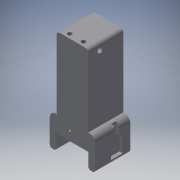
# Autodesk Inventor part: Part1
Saved by Autodesk Inventor 2016 (Build 200138000, 138)
## iProperties
Created: 2016-11-19
Part Number: Part1
Material: Generic
Document SubType Name: Modeling
Designer: Juraj
Density: 1 g/cm^3
Appearance: Default
Author: Juraj
Autodesk Inventor part; units mm, degrees
ref_plane "YZ Plane" through (0, 0, 0) normal (1, 0, 0) x (0, 1, 0)
ref_plane "XZ Plane" through (0, 0, 0) normal (0, 1, 0) x (-1, 0, 0)
ref_plane "XY Plane" through (0, 0, 0) normal (0, 0, 1) x (1, 0, 0)
sketch "Sketch1" plane through (0, 0, 0) normal (0, 1, 0) x (-1, 0, 0)
  line L0 (7.9968, 14.4905) -> (-11.0032, 14.4905)
  line L1 (-11.0032, 14.4905) -> (-11.0032, -38.5095)
  line L2 (-11.0032, -38.5095) -> (7.9968, -38.5095)
  line L3 (7.9968, -38.5095) -> (7.9968, 14.4905)
  point P0 (0, 0)
  dimension "d0" = 19
  dimension "d1" = 53
  constraints: 8 end point, 2 parallel, 1 horizontal, 1 perpendicular
  measures "d0" distance of L0.start L0.end
  measures "d1" distance of L2.end L0.start
extrude "Extrusion1" add sketch "Sketch1" along normal blind 1
sketch "Sketch2" plane through (0, 1, 0) normal (0, 1, 0) x (1, 0, 0)
  line L0 (9.0032, -13.4905) -> (-5.9968, -13.4905)
  line L1 (-5.9968, -13.4905) -> (-5.9968, 37.5095)
  line L2 (-5.9968, 37.5095) -> (9.0032, 37.5095)
  line L3 (9.0032, 37.5095) -> (9.0032, -13.4905)
  line L4 (11.0032, -14.4905) -> (11.0032, 38.5095) projected
  line L5 (-7.9968, -14.4905) -> (11.0032, -14.4905) projected
  line L6 (-7.9968, 38.5095) -> (-7.9968, -14.4905) projected
  line L7 (11.0032, 38.5095) -> (-7.9968, 38.5095) projected
  point P0 (0, 0)
  dimension "d4" = 2
  dimension "d5" = 1
  dimension "d6" = 2
  dimension "d7" = 1
  constraints: 8 end point, 2 parallel, 1 horizontal, 1 perpendicular
  measures "d4" distance between parallel lines of L4 L3
  measures "d5" distance between parallel lines of L5 L0
  measures "d6" distance between parallel lines of L6 L1
  measures "d7" distance between parallel lines of L7 L2
extrude "Extrusion2" add sketch "Sketch2" along normal blind 18
sketch "Sketch5" plane through (11.0032, 0, -38.5095) normal (0, 0, -1) x (-1, 0, 0)
  line L0 (17, 1) -> (2, 1) projected
  line L1 (9.5, 1) -> (9.5, 6)
  line L2 (9.5, 6) -> (9.5, 13.4)
  circle A0 centre (9.5, 13.4) radius 2
  line L3 (2, 1) -> (2, 19) projected
  line L4 (17, 1) -> (17, 19) projected
  point P0 (11.0032, 0)
  dimension "d28" = 5
  dimension "d29" = 7.4
  dimension "d30" = 4
  dimension "d31" = 7.5
  dimension "d32" = 7.5
  constraints: 4 end point, 1 centre point, 1 coincident, 1 midpoint, 1 perpendicular, 1 vertical
  measures "d28" distance of L1.start L1.end
  measures "d29" distance of L1.end L2.end
  measures "d30" diameter of A0
  measures "d31" distance between parallel lines of L3 L1
  measures "d32" distance between parallel lines of L4 L1
extrude "Extrusion3" cut sketch "Sketch5" against normal blind 13
sketch "Sketch6" plane through (-5.9968, 1, -37.5095) normal (0, 0, 1) x (1, 0, 0)
  circle A0 centre (7.5, 12.4) radius 2 projected
  circle A1 centre (7.5, 12.4) radius 3.55
  line L0 (3.9514, 12.5) -> (0, 12.5)
  line L1 (0, 0) -> (0, 18) projected
  line L2 (11.0486, 12.5) -> (15, 12.5)
  line L3 (15, 0) -> (15, 18) projected
  line L4 (15, 12.5) -> (15, 0)
  line L5 (15, 0) -> (0, 0) projected
  line L6 (15, 0) -> (0, 0)
  line L7 (0, 0) -> (0, 12.5)
  line L8 (3.9514, 12.5) -> (0, 12.5)
  line L9 (0, 12.5) -> (0, 18)
  line L10 (0, 18) -> (3.9514, 18)
  line L11 (3.9514, 18) -> (3.9514, 12.5)
  line L12 (11.0486, 12.5) -> (15, 12.5)
  line L13 (15, 12.5) -> (15, 18)
  line L14 (15, 18) -> (11.0486, 18)
  line L15 (11.0486, 18) -> (11.0486, 12.5)
  point P0 (5.9968, -1)
  dimension "d35" = 7.1
  constraints: 26 end point, 4 parallel, 4 point on line, 3 collinear, 3 horizontal, 2 perpendicular, 2 point on circle, 1 centre point, 1 coincident
  measures "d35" diameter of A1
extrude "Extrusion4" add sketch "Sketch6" along normal blind 3.5 contours A1 L2 L3 L5 L1 L0 | L15 L14 L3 L2 | L0 L1 L10 L11
sketch "Sketch7" plane through (9.0032, 1, 13.4905) normal (0, 0, -1) x (-1, 0, 0)
  circle A0 centre (7.5, 12.4) radius 2 projected
  circle A1 centre (7.5, 12.4) radius 2
  line L0 (15, 0) -> (0, 0) projected
  line L1 (0, 0) -> (15, 0)
  line L2 (15, 0) -> (15, 18) projected
  circle A2 centre (7.5, 12.4) radius 3.55
  line L3 (11.0486, 12.5) -> (15, 12.5)
  line L4 (15, 12.5) -> (15, 0)
  line L5 (17, -1) -> (-2, -1) projected
  line L6 (15, 0) -> (0, 0)
  line L7 (0, 0) -> (0, 12.5)
  line L8 (0, 12.5) -> (3.9514, 12.5)
  line L9 (0, 18) -> (15, 18) projected
  line L10 (3.9514, 12.5) -> (0, 12.5)
  line L11 (0, 12.5) -> (0, 18)
  line L12 (0, 18) -> (3.9514, 18)
  line L13 (3.9514, 18) -> (3.9514, 12.5)
  line L14 (11.0486, 12.5) -> (15, 12.5)
  line L15 (15, 12.5) -> (15, 18)
  line L16 (15, 18) -> (11.0486, 18)
  line L17 (11.0486, 18) -> (11.0486, 12.5)
  point P0 (9.0032, -1)
  dimension "d40" = 7.1
  constraints: 28 end point, 5 equal length, 5 perpendicular, 3 horizontal, 2 centre point, 2 coincident, 2 point on circle, 2 point on line
  measures "d40" diameter of A2
extrude "Extrusion5" add sketch "Sketch7" along normal blind 3.5 contours L0 L7 L8 A2 L3 L2 | L3 L17 L9 L2 | L11 L9 L13 L8
sketch "Sketch9" plane through (0, 1, 0) normal (0, 1, 0) x (1, 0, 0)
  line L0 (-5.9968, -9.9905) -> (9.0032, -9.9905) projected
  line L1 (9.0032, -9.9905) -> (9.0032, -7.9905)
  line L2 (9.0032, -9.9905) -> (9.0032, 34.0095) projected
  line L3 (9.0032, -7.9905) -> (-5.9968, -7.9905)
  line L4 (-5.9968, 34.0095) -> (-5.9968, -9.9905) projected
  line L5 (9.0032, 34.0095) -> (9.0032, 33.0095)
  line L6 (9.0032, 33.0095) -> (-5.9968, 33.0095)
  line L7 (-5.9968, 33.0095) -> (-5.9968, 34.0095)
  line L8 (9.0032, 34.0095) -> (-5.9968, 34.0095)
  line L9 (-5.9968, 33.0095) -> (-5.9968, 34.0095)
  line L10 (9.0032, 34.0095) -> (5.0518, 34.0095) projected
  line L11 (9.0032, 34.0095) -> (-5.9968, 34.0095)
  line L12 (-5.9968, -13.4905) -> (-5.9968, 37.5095) projected
  point P0 (0, 0)
  dimension "d46" = 2
  dimension "d47" = 1
  constraints: 16 end point, 4 point on line, 3 perpendicular, 2 collinear, 1 horizontal
  measures "d46" distance of L0.end L1.end
  measures "d47" distance of L2.end L5.end
extrude "Extrusion7" add sketch "Sketch9" along normal blind 18 contours L4 L3 L1 L0 | L4 L8 L2 L6
sketch "Sketch12" plane through (0, 1, 0) normal (0, 1, 0) x (1, 0, 0)
  line L0 (9.0032, 33.0095) -> (-5.9968, 33.0095) projected
  line L1 (-5.9968, -7.9905) -> (-4.6968, -7.9905)
  line L2 (-4.6968, -7.9905) -> (-4.6968, 33.0095)
  line L3 (-5.9968, 33.0095) -> (-5.9968, -7.9905) projected
  line L4 (-5.9968, -7.9905) -> (-5.9968, 33.0095)
  line L5 (-5.9968, 33.0095) -> (-4.6968, 33.0095)
  line L6 (-5.9968, 33.0095) -> (-4.6968, 33.0095)
  line L7 (5.0518, 34.0095) -> (-2.0454, 34.0095) projected
  line L8 (9.0032, -7.9905) -> (7.7032, -7.9905)
  line L9 (7.7032, -7.9905) -> (7.7032, 33.0095)
  line L10 (-5.9968, 33.0095) -> (9.0032, 33.0095) projected
  line L11 (9.0032, 33.0095) -> (7.7032, 33.0095)
  line L12 (9.0032, 33.0095) -> (9.0032, -7.9905) projected
  line L13 (9.0032, -7.9905) -> (9.0032, 33.0095)
  line L14 (9.0032, 33.0095) -> (7.7032, 33.0095)
  point P0 (0, 0)
  point P1 (31.8085, 33.0095)
  point P2 (9.0032, 34.0095)
  point P3 (-5.9968, 34.0095)
  dimension "d61" = 1.3
  dimension "d153" = 1.3
  constraints: 20 end point, 4 perpendicular, 3 point on line, 2 collinear, 1 vertical
  measures "d61" distance of L1.start L1.end
  measures "d153" distance between parallel lines of L12 L9
extrude "Extrusion9" add sketch "Sketch12" along normal blind 18
sketch "Sketch10" plane through (9.0032, 19, -34.0095) normal (0, 0, -1) x (-1, 0, 0)
  circle A0 centre (7.5, -5.6) radius 2 projected
  circle A1 centre (7.5, -5.6) radius 2
  point P0 (9.0032, -19)
  constraints: 1 centre point, 1 coincident
extrude "Extrusion8" cut sketch "Sketch10" against normal blind 46
sketch "Sketch13" plane through (0, 1, 0) normal (0, 1, 0) x (1, 0, 0)
  line L0 (3.5032, -6.9905) -> (-0.4968, -6.9905)
  line L1 (-4.6968, -7.9905) -> (-4.6968, 33.0095) projected
  line L2 (-4.6968, 19.3095) -> (-3.1968, 19.3095)
  line L3 (-3.1968, 19.3095) -> (-3.1968, 21.3095)
  line L4 (-3.1968, 21.3095) -> (-4.6968, 21.3095)
  line L5 (7.7032, 19.3095) -> (6.2032, 19.3095)
  line L6 (6.2032, 19.3095) -> (6.2032, 21.3095)
  line L7 (6.2032, 21.3095) -> (7.7032, 21.3095)
  line L8 (-0.4968, -7.9905) -> (3.5032, -7.9905) projected
  line L9 (3.5032, -7.9905) -> (3.5032, -6.9905)
  line L10 (-0.4968, -7.9905) -> (-0.4968, -6.9905)
  line L11 (3.5032, -7.9905) -> (-0.4968, -7.9905)
  line L12 (7.7032, -7.9905) -> (-4.6968, -7.9905) projected
  line L13 (7.7032, 19.3095) -> (7.7032, 21.3095)
  line L14 (7.7032, 33.0095) -> (7.7032, -7.9905) projected
  point P0 (0, 0)
  dimension "d76" = 26.3
  dimension "d77" = 2
  dimension "d78" = 1.5
  dimension "d79" = 1.5
  dimension "d89" = 1
  dimension "d169" = 0
  dimension "d170" = 2
  constraints: 22 end point, 5 perpendicular, 5 point on line, 2 collinear, 1 parallel
  measures "d76" distance between parallel lines of L0 L5
  measures "d77" distance of L5.end L6.end
  measures "d78" distance of L3.end L4.end
  measures "d79" distance of L6.end L7.end
  measures "d89" distance of L8.end L0.start
  measures "d169" distance between parallel lines of L14 L13
  measures "d170" distance of L5.start L7.end
extrude "Extrusion10" add sketch "Sketch13" along normal blind 8
sketch "Sketch11" plane through (0, 1, 0) normal (0, 1, 0) x (1, 0, 0)
  line L0 (7.5032, -6.9905) -> (-4.4968, -6.9905)
  line L1 (-4.4968, -6.9905) -> (-4.4968, 19.0095)
  line L2 (-4.4968, 19.0095) -> (7.5032, 19.0095)
  line L3 (7.5032, 19.0095) -> (7.5032, -6.9905)
  line L4 (-5.9968, -7.9905) -> (-5.9968, 33.0095) projected
  line L5 (1.5032, 19.0095) -> (5.5033, 19.0095)
  line L6 (5.5033, 19.0095) -> (5.5033, 28.0095)
  line L7 (5.5033, 28.0095) -> (-2.4967, 28.0095)
  line L8 (-2.4967, 28.0095) -> (-2.4967, 19.0095)
  line L9 (5.5033, 23.0095) -> (-2.4967, 23.0095)
  line L10 (-2.4967, 23.0095) -> (-2.4967, 32.0095)
  line L11 (-2.0454, 37.5095) -> (-2.0454, 34.0095) projected
  line L12 (9.0032, -7.9905) -> (-5.9968, -7.9905) projected
  line L13 (3.5032, -6.9905) -> (-0.4968, -6.9905) projected
  point P0 (0, 0)
  point P1 (-2.0468, 37.5095)
  point P2 (-2.0468, 34.0095)
  dimension "d52" = 12
  dimension "d53" = 1.5
  dimension "d54" = 9
  dimension "d55" = 8
  dimension "d56" = 4
  dimension "d57" = 9
  dimension "d59" = 26
  dimension "d83" = 0
  constraints: 20 end point, 5 perpendicular, 4 point on line, 2 horizontal, 2 vertical, 1 midpoint, 1 other
  measures "d52" distance of L0.start L0.end
  measures "d53" distance between parallel lines of L4 L1
  measures "d54" distance of L5.end L6.end
  measures "d55" distance of L6.end L7.end
  measures "d56" distance between parallel lines of L2 L9
  measures "d57" distance of L9.end L10.end
  measures "d59" distance of L0.end L1.end
  measures "d83" distance between parallel lines of L13 L0
fillet "Fillet1" radius 2 2 edges at (-0.4968, 9, 7.4905) (3.5032, 9, 7.4905)
fillet "Fillet2" radius 0.5 2 edges at (6.2032, 9, -20.3095) (-3.1968, 9, -20.3095)
sketch "Sketch16" plane through (11.0032, 0, 14.4905) normal (1, 0, 0) x (0, 0, -1)
  circle A0 centre (4, 7) radius 1.5
  line L0 (53, 0) -> (0, 0) projected
  line L1 (0, 0) -> (0, 19) projected
  point P0 (14.4905, 0)
  point P1 (52, 0)
  dimension "d84" = 3
  dimension "d85" = 7
  dimension "d86" = 4
  constraints: 1 centre point
  measures "d84" diameter of A0
  measures "d85" distance from line of L0 A0.centre
  measures "d86" distance from line of L1 A0.centre
extrude "Extrusion12" cut sketch "Sketch16" against normal blind 19
sketch "Sketch20" plane through (11.0032, 0, 14.4905) normal (1, 0, 0) x (0, 0, -1)
  line L0 (0, 19) -> (53, 19) projected
  line L1 (43, 19) -> (62, 19)
  line L2 (62, 19) -> (62, 0)
  line L3 (62, 0) -> (43, 0)
  line L4 (43, 0) -> (43, 19)
  line L5 (53, 15.4) -> (53, 11.4) projected
  line L6 (53, 0) -> (53, 19) projected
  point P0 (14.4905, 0)
  dimension "d106" = 9
  dimension "d107" = 10
  constraints: 8 end point, 2 parallel, 1 horizontal, 1 perpendicular, 1 point on line
  measures "d106" distance between parallel lines of L5 L2
  measures "d107" distance between parallel lines of L6 L4
extrude "Extrusion15" add sketch "Sketch20" along normal blind 4
sketch "Sketch21" plane through (-7.9968, 0, -38.5095) normal (-1, 0, 0) x (0, 0, 1)
  line L0 (-9, 0) -> (-9, 19) projected
  line L1 (-9, 19) -> (-9, 0)
  line L2 (0, 0) -> (0, 19) projected
  line L3 (10, 0) -> (10, 19) projected
  line L4 (-9, 19) -> (10, 19)
  line L5 (53, 0) -> (10, 0) projected
  line L6 (10, 19) -> (10, 0)
  line L7 (10, 0) -> (-9, 0)
  line L8 (0, 0) -> (-9, 0) projected
  point P0 (38.5095, 0)
  point P1 (4.5, 20)
  dimension "d113" = 9
  constraints: 8 end point, 1 collinear, 1 horizontal, 1 perpendicular
  measures "d113" distance between parallel lines of L0 L2
extrude "Extrusion16" add sketch "Sketch21" along normal blind 4
fillet "Fillet5" radius 3.5 2 edges at (15.0032, 9.5, -28.5095) (-11.9968, 9.5, -28.5095)
sketch "Sketch22" plane through (-11.9968, 0, -38.5095) normal (-1, 0, 0) x (0, 0, 1)
  line L0 (-7, 15.5) -> (3, 15.5)
  line L1 (3, 8.5) -> (-7, 8.5)
  line L2 (-7, 8.5) -> (-7, 15.5)
  line L3 (6.5, 19) -> (-9, 19) projected
  line L4 (-9, 0) -> (6.5, 0) projected
  line L5 (-9, 19) -> (-9, 0) projected
  line L6 (3, 15.5) -> (3, 8.5)
  line L7 (10, 0) -> (10, 19) projected
  line L8 (3, 12) -> (3, 13.5)
  line L9 (3, 13.5) -> (10, 13.5)
  line L10 (10, 0) -> (10, 19) projected
  line L11 (3, 12) -> (3, 10.5)
  line L12 (3, 10.5) -> (10, 10.5)
  point P0 (38.5095, 0)
  dimension "d114" = 10
  dimension "d132" = 2
  dimension "d133" = 3
  dimension "d151" = 2
  dimension "d152" = 5.5
  constraints: 16 end point, 4 point on line, 2 perpendicular, 1 horizontal, 1 midpoint, 1 parallel
  measures "d114" distance of L0.start L0.end
  measures "d132" distance between parallel lines of L0 L9
  measures "d133" distance between parallel lines of L9 L12
  measures "d151" distance between parallel lines of L1 L12
  measures "d152" distance between parallel lines of L3 L9
extrude "Extrusion17" cut sketch "Sketch22" against normal blind 2
sketch "Sketch23" plane through (-9.9968, 0, -38.5095) normal (-1, 0, 0) x (0, 0, 1)
  circle A0 centre (8.1623, 12) radius 1.5
  line L0 (9.6623, 13.5) -> (6.5, 13.5) projected
  line L1 (9.6623, 13.5) -> (9.6623, 10.5) projected
  point P0 (38.5095, 0)
  dimension "d126" = 3
  dimension "d127" = 1.5
  dimension "d128" = 1.5
  constraints: 1 centre point
  measures "d126" diameter of A0
  measures "d127" distance from line of L0 A0.centre
  measures "d128" distance from line of A0.centre L1
extrude "Extrusion18" cut sketch "Sketch23" against normal blind 5 contours A0
sketch "Sketch24" plane through (15.0032, 0, 14.4905) normal (1, 0, 0) x (0, 0, -1)
  line L0 (60, 16.5) -> (50, 16.5)
  line L1 (50, 16.5) -> (50, 9.5)
  line L2 (50, 9.5) -> (60, 9.5)
  line L3 (60, 9.5) -> (60, 16.5)
  line L4 (62, 19) -> (46.5, 19) projected
  line L5 (46.5, 0) -> (62, 0) projected
  line L6 (50, 14.5) -> (43.0172, 14.5)
  line L7 (46.5, 19) -> (46.5, 13.5) projected
  line L8 (50, 11.5) -> (43.0172, 11.5)
  line L9 (43.0172, 14.5) -> (43.0172, 11.5)
  line L10 (43, 0) -> (43, 19) projected
  point P0 (14.4905, 0)
  point P1 (62, 20)
  point P2 (49.3544, 14.5)
  dimension "d137" = 10
  dimension "d150" = 2
  constraints: 14 end point, 3 parallel, 2 horizontal, 2 perpendicular, 2 point on line, 1 other
  measures "d137" distance of L0.start L0.end
  measures "d150" distance between parallel lines of L8 L2
extrude "Extrusion19" cut sketch "Sketch24" against normal blind 2
sketch "Sketch25" plane through (13.0032, 0, 14.4905) normal (1, 0, 0) x (0, 0, -1)
  arc A0 (44.8377, 10.5) -> (44.8377, 13.5) centre (44.8377, 12) ccw projected
  circle A1 centre (44.8377, 12) radius 1.5
  point P0 (14.4905, 0)
  constraints: 1 centre point, 1 coincident
extrude "Extrusion20" cut sketch "Sketch25" against normal blind 5
sketch "Sketch28" plane through (0, 19, 0) normal (0, 1, 0) x (1, 0, 0)
  circle A0 centre (-8.3468, 34.5095) radius 1.25
  line L0 (11.0032, 38.5095) -> (-7.9968, 38.5095) projected
  line L1 (-4.6968, -7.9905) -> (-4.6968, 33.0095) projected
  line L2 (-11.9968, 32.0095) -> (-11.9968, 47.5095) projected
  line L3 (11.0032, 38.5095) -> (-7.9968, 38.5095) projected
  line L4 (1.5032, 38.5095) -> (1.5032, 41.4251)
  circle A1 centre (11.3532, 34.5095) radius 1.25
  circle A2 centre (-4.9968, -11.8434) radius 1.25
  line L5 (-7.9968, 28.5095) -> (-7.9968, -14.4905) projected
  line L6 (-2.0454, -13.4905) -> (-2.0454, -9.9905) projected
  circle A3 centre (8.0032, -11.8434) radius 1.25
  point P0 (0, 0)
  dimension "d154" = 2.5
  dimension "d155" = 4
  dimension "d156" = 3.65
  dimension "d157" = 3.65
  dimension "d158" = 2.5
  dimension "d159" = 3
  dimension "d160" = 2.9514
  constraints: 4 centre point, 2 end point, 2 symmetric about line, 1 midpoint, 1 vertical, 2 other
  measures "d154" diameter of A0
  measures "d155" distance from line of L0 A0.centre
  measures "d156" distance from line of L1 A0.centre
  measures "d157" distance from line of L2 A0.centre
  measures "d158" diameter of A2
  measures "d159" distance from line of L5 A2.centre
  measures "d160" distance from line of L6 A2.centre
extrude "Extrusion21" cut sketch "Sketch28" against normal blind 10
sketch "Sketch29" plane through (-7.9968, 0, 14.4905) normal (0, 0, 1) x (1, 0, 0)
  circle A0 centre (13.6, 2.5) radius 1.25
  line L0 (11.5, 1) -> (11.5, 7) projected
  line L1 (15.7, 19) -> (15.7, 1) projected
  line L2 (15.7, 1) -> (3.3, 1) projected
  line L3 (9.5, 1) -> (9.5, 3.9064)
  circle A1 centre (5.4, 2.5) radius 1.25
  point P0 (7.9968, 0)
  dimension "d163" = 2.5
  dimension "d164" = 2.1
  dimension "d165" = 2.1
  dimension "d166" = 1.5
  constraints: 2 centre point, 2 end point, 1 midpoint, 1 symmetric about line, 1 vertical, 1 other
  measures "d163" diameter of A0
  measures "d164" distance from line of A0.centre L0
  measures "d165" distance from line of L1 A0.centre
  measures "d166" distance from line of L2 A0.centre
extrude "Extrusion22" cut sketch "Sketch29" against normal blind 10
fillet "Fillet6" radius 2 2 edges at (-7.9968, 9.5, 14.4905) (11.0032, 9.5, 14.4905)
fillet "Fillet7" radius 1.5 4 edges at (11.0032, 9.5, -47.5095) (-7.9968, 9.5, -47.5095) (15.0032, 9.5, -47.5095) (-11.9968, 9.5, -47.5095)
sketch "Sketch30" plane through (0, 19, 0) normal (0, 1, 0) x (1, 0, 0)
  line L0 (-6.9968, -12.4905) -> (-6.9968, 29.5095)
  line L1 (-6.9968, 29.5095) -> (-8.4968, 29.5095)
  line L2 (-7.9968, 46.0095) -> (-7.9968, 38.5095) projected
  line L3 (-7.9968, 38.5095) -> (-7.9968, 46.0095)
  arc A0 (-7.9968, 46.0095) -> (-9.4968, 47.5095) centre (-9.4968, 46.0095) ccw projected
  arc A1 (-7.9968, 46.0095) -> (-9.4968, 47.5095) centre (-9.4968, 46.0095) ccw
  line L4 (-9.4968, 47.5095) -> (-10.4968, 47.5095) projected
  line L5 (-9.4968, 47.5095) -> (-10.4968, 47.5095)
  line L6 (-11.9968, 46.0095) -> (-11.9968, 32.0095) projected
  arc A2 (-10.4968, 47.5095) -> (-11.9968, 46.0095) centre (-10.4968, 46.0095) ccw
  arc A3 (-11.9968, 32.0095) -> (-8.4968, 28.5095) centre (-8.4968, 32.0095) ccw projected
  line L7 (-11.9968, 46.0095) -> (-11.9968, 32.0095)
  arc A4 (-10.9968, 32.0095) -> (-8.4968, 29.5095) centre (-7.6108, 32.8955) ccw
  line L8 (-7.9968, 28.5095) -> (-7.9968, -12.4905) projected
  line L9 (-7.9968, 28.5095) -> (-8.4968, 28.5095) projected
  line L10 (-7.9968, 28.5095) -> (-8.4968, 28.5095) projected
  arc A5 (-11.9968, 32.0095) -> (-8.4968, 28.5095) centre (-8.4968, 32.0095) ccw
  line L11 (-8.4968, 28.5095) -> (-7.9968, 28.5095)
  line L12 (-7.9968, 28.5095) -> (-7.9968, -12.4905)
  arc A6 (-6.9968, -12.4905) -> (-5.8853, -13.4905) centre (-5.7634, -12.2372) ccw
  arc A7 (-7.9968, -12.4905) -> (-5.9968, -14.4905) centre (-5.9968, -12.4905) ccw projected
  arc A8 (-7.9968, -12.4905) -> (-5.9968, -14.4905) centre (-6.0394, -12.533) ccw
  line L13 (-5.9968, -14.4905) -> (1.5032, -14.4905)
  line L14 (1.5032, -14.4905) -> (1.5032, -16.2241)
  line L15 (-10.9968, 37.5095) -> (-10.9968, 32.0095)
  line L16 (-5.8853, -13.4905) -> (1.5032, -13.4905)
  line L17 (5.0532, -13.4905) -> (-2.0468, -13.4905) projected
  line L18 (-10.9968, 37.5095) -> (1.5032, 37.5095)
  line L19 (-7.9968, 38.5095) -> (1.5032, 38.5095)
  line L20 (10.0032, -12.4905) -> (10.0032, 29.5095)
  line L21 (10.0032, 29.5095) -> (11.5032, 29.5095)
  line L22 (11.0032, 38.5095) -> (11.0032, 46.0095)
  arc A9 (12.5032, 47.5095) -> (11.0032, 46.0095) centre (12.5032, 46.0095) ccw
  line L23 (12.5032, 47.5095) -> (13.5032, 47.5095)
  line L24 (15.0032, 46.0095) -> (15.0032, 32.0095)
  arc A10 (15.0032, 46.0095) -> (13.5032, 47.5095) centre (13.5032, 46.0095) ccw
  arc A11 (11.5032, 28.5095) -> (15.0032, 32.0095) centre (11.5032, 32.0095) ccw
  arc A12 (11.5032, 29.5095) -> (14.0032, 32.0095) centre (10.6172, 32.8955) ccw
  line L25 (11.0032, 28.5095) -> (11.0032, -12.4905)
  line L26 (11.0032, 28.5095) -> (11.5032, 28.5095)
  arc A13 (8.8916, -13.4905) -> (10.0032, -12.4905) centre (8.7697, -12.2372) ccw
  arc A14 (9.0032, -14.4905) -> (11.0032, -12.4905) centre (9.0032, -12.4905) ccw
  line L27 (9.0032, -14.4905) -> (1.5032, -14.4905)
  line L28 (14.0032, 37.5095) -> (14.0032, 32.0095)
  line L29 (8.8916, -13.4905) -> (1.5032, -13.4905)
  line L30 (14.0032, 37.5095) -> (1.5032, 37.5095)
  line L31 (11.0032, 38.5095) -> (1.5032, 38.5095)
  circle A15 centre (11.3532, 34.5095) radius 1.25 projected
  circle A16 centre (11.3532, 34.5095) radius 1.25
  circle A17 centre (-8.3468, 34.5095) radius 1.25 projected
  circle A18 centre (-8.3468, 34.5095) radius 1.25
  circle A19 centre (8.0032, -11.8434) radius 1.25 projected
  circle A20 centre (8.0032, -11.8434) radius 1.25
  circle A21 centre (-4.9968, -11.8434) radius 1.25 projected
  circle A22 centre (-4.9968, -11.8434) radius 1.25
  point P0 (0, 0)
  point P1 (5.0518, -13.4905)
  point P2 (-2.0454, -13.4905)
  point P3 (-2.0454, 37.5095)
  point P4 (5.0518, 37.5095)
  dimension "d182" = 2.5
  dimension "d173" = 3.5
  dimension "d175" = 1
  dimension "d176" = 1
  dimension "d177" = 3.5
  dimension "d178" = 0
  constraints: 50 end point, 24 point on circle, 22 symmetric about line, 15 centre point, 4 coincident, 4 vertical, 3 collinear, 2 concentric, 2 tangent, 1 horizontal, 1 midpoint, 9 other
  measures "d173" radius of A4
  measures "d175" distance between parallel lines of L8 L0
  measures "d176" distance between parallel lines of L9 L1
  measures "d177" radius of A3
  measures "d178" horizontal distance of L1.end L9.end
extrude "Extrusion23" add sketch "Sketch30" along normal blind 2 contours L2 L19 L31 L22 A9 L23 A10 L24 A11 L26 L25 A14 L27 L13 A7 L8 L9 A3 L6 A2 L4 A0 | A7 A8
equation "\"d6\" = d4"
equation "\"d7\" = d5"
equation "\"d153\" = d61"
equation "\"d78\" = d79"
equation "\"d173\" = d177"
equation "\"d175\" = d179"
equation "\"d176\" = d179"
equation "\"d179\" = 1"
body "Solid1"
